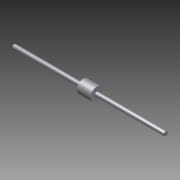
# Autodesk Inventor part: 042-DXDE0_rod
Saved by Autodesk Inventor 2012 (Build 160160000, 160)
## iProperties
Created: 2013-01-17
Part Number: 042-DXDE0_rod
Material: Default
Catalog Web Link: www.cadenas.de
Description: Standard Air Cylinder_rod-Original Line - Standard Air Cylinders
Vendor: BIMBA
Document SubType Name: Modeling
Designer: William
Manufacturer: BIMBA
Density: 1 g/cm^3
Category: PARTsolutions
Company: BIMBA
Title: 042-DXDE0_rod
Author: Cadenas PARTsolutions
Comments: Original Line - Standard Air Cylinders
PSOL_IDENT_0: {\\10.0.0.242\data_v9\23d-libs\bimba\bimba\bimba_imperial\bimba_full_line\original_line_cylinders\st
PSOL_IDENT_1: andard_air_cylinders\rod.prj},280 {VTYP=3D},{NB=042-DXDE0_rod},{LINA=042-DXDE0_rod},{NN=Standard Air
PSOL_IDENT_2: Cylinder_rod},{DATE=11.09.2012 07:37:40},{GEOMDATE=06.09.2012 09:06:00},{VERSION=},{LINEID=50},{LIN
PSOL_IDENT_3: ESUBID=-1},{WBVAR=STROKE,ACTING,MNT,DER,NR,BM,CO,M,EE,EEL,K,Q,Y,F,G,T,B,H,SER,SR,NT,W,E,HL,ST,STP,PR
PSOL_IDENT_4: C,PB,COLOR1}  {NB=042-DXDE0_rod},{LINA=042-DXDE0_rod},{KT=DUMMY},{PN=042-DXDE},{DASH=-},{BORE=0.7500
PSOL_IDENT_5: 0000},{BOREPN=04},{STROKE=2.000},{STROKEALG=[0.001:50/0.001]},{STROKE1=2.000},{ACTING=D},{ACTINGALG=
PSOL_IDENT_6: '' , 'Single Acting' , 'R' , 'Reverse Single Acting' , 'D' , 'Double Acting' },{ACTINGPN=D},{MNT=X}
PSOL_IDENT_7: ,{MNTALG= '' , 'Front Nose Mounting' , 'P' , 'Rear Pivot Mounting' , 'XP' , 'Double End or Pivot Mou
PSOL_IDENT_8: nting' , 'X' , 'Double End Mounting' , 'BF' , 'Front Block Mounting' , 'BR' , 'Rear Block Mounting f
PSOL_IDENT_9: or Vertical Positioning' , 'BFT' , 'Front Block Trunnion Mounting' , 'BRT' , 'Rear Block Trunnion Mo
PSOL_IDENT_10: unting' },{TYPE=},{MNTPN=X},{DER=DE},{DERALG= 'DE' , 'With Double End Rod' },{NR=},{NRALG= '' , 'N/A
PSOL_IDENT_11: ' },{NRPN=},{BM=},{BMALG= '' , 'N/A' },{BMPN=},{CO=},{COALG= '' , 'N/A' },{M=},{MALG= '', 'Without M
PSOL_IDENT_12: agnet', 'M', 'With Magnet' },{EE=},{EEL=0},{EEMAX=48},{EEALG= '', 'Without Extra Extension', 'EE', '
PSOL_IDENT_13: With Extra Extension' },{EELALG=0},{EEPN=},{EEPN1=0.000},{K=},{KALG= '', 'Standard' , 'K' , 'Ports R
PSOL_IDENT_14: otated 90deg' },{KPN=},{Q=},{QALG= '' , 'Without Side Ported Rear Head' , 'Q' , 'With Side Ported Re
PSOL_IDENT_15: ar Head' },{QPN=},{Y=},{YALG= '' , 'N/A' },{YPN=},{F=},{FALG= '', 'Standard', 'F', 'Molycoated Body'
PSOL_IDENT_16: },{FPN=},{G=},{GPN=},{T=},{TALG= '' , 'Standard' , 'N' , 'Low Temperature' , 'V' , 'High Temperatur
PSOL_IDENT_17: e' },{NPN=},{VPN=},{B=},{BALG= '', 'Without Bumper' , 'B' , 'With Bumper' },{BPN=},{H=},{HALG= '', '
PSOL_IDENT_18: N/A' },{HPN=},{SER=},{SERALG= '' , 'Without Spring Return' , 'JS' , 'With Spring Return' },{SR=},{SR
PSOL_IDENT_19: ALG= 'C' , 'Carbon Steel Rod' , 'SR' , '303 Stainless Steel Rod' , '' , '303 Stainless Steel Rod1' }
PSOL_IDENT_20: ,{SRPN=},{SRCON=0},{NT=},{NTPN=},{W=},{WALG= '' , 'Without Wiper' , 'W' , 'With Wiper' },{WPN=},{E=}
PSOL_IDENT_21: ,{EALG= '' , 'Without Special Lube and Seals' , 'E' , 'With Special Lube and Seals' },{EPN=},{HL=},{
PSOL_IDENT_22: HLALG= '' , 'Wihout Low Pressure Hydraulic' , 'HL' , 'With Low Pressure Hydraulic' },{ST=},{STALG= '
PSOL_IDENT_23: ' , 'Without Switch Track' , 'T' , 'With Switch Track' },{STP=},{STPALG= '' , 'N/A' },{STPN=},{PRC=}
PSOL_IDENT_24: ,{PRCALG= '' , 'Without Piston Rod Clevis' , 'D-166-1' , 'With Piston Rod Clevis' },{PRCPN=},{PB=},{
PSOL_IDENT_25: PBALG= '' , 'Without Pivot Bracket' , 'D-167' , 'With Pivot Bracket' },{PBPN=},{TLEN=3.2570},{TEXT=0
PSOL_IDENT_26: .233333},{SPACE=0.133333},{FRAC=9.0000},{RGCON=},{RGDACCON=R},{RHCON=DX},{RHCONON=0},{RHACCON=},{FNU
PSOL_IDENT_27: TCON=1},{RNUTCON=1},{FNUTPN=D-9},{RNUTPN=D-9},{FNUTTRANS=0.0000},{RNUTTRANS=0.0000},{VHOLECON=0},{A1
PSOL_IDENT_28: =1.5940},{A1N=0.8750},{A1P=1.5940},{A1B=1.5940},{A4=0.2525},{A4N=0.3130},{A4P=0.2525},{A5=0.0300},{A
PSOL_IDENT_29: 1H=1.594},{A1NH=0.5310},{A1PH=1.5940},{A1BH=1.0940},{A1SH=1.2190},{A2H=0.2190},{A2NH=0.2190},{LENGTH
PSOL_IDENT_30: =4.0000},{LENGTH1=4.0000},{LENGTH2=0.0000},{MUL=2.0000},{MUL11=2.0000},{MUL22=5.3800},{MUL33=5.3800}
PSOL_IDENT_31: ,{MUL2=2.0000},{MUL211=2.0000},{MUL222=2.6900},{MUL233=2.6900},{SSS=4.0000},{RGLEN=1.3715},{RHLEN=1.
PSOL_IDENT_32: 3715},{SSS1=3.0000},{A13=1.3120},{THDLEN1=0.5000},{THD1=0.2500},{TAB=UNF},{THDLEN=0.5000},{THD=0.250
PSOL_IDENT_33: 0},{OD=0.7615},{RODL=4.9060},{PL=0.8120},{RODDIA=0.2500},{HEX=0.2500},{RODTRANS=2.0000},{G1=0.1250},
PSOL_IDENT_34: {ON=0},{G5=0.6250},{DERLEN=4.0940},{THOLE=0.0000},{WF=0.2200},{BADD=0.0000},{MADD=0.0000},{NVADD=0.0
PSOL_IDENT_35: 00},{JRADD=0.00000},{COLOR=0.71,0.71,0.71,0.00},{GROOVE=1},{HOL=0},{D7=0.2520},{H1=1.1175},{D1=0.862
PSOL_IDENT_36: 5},{D1RH=0.8625},{D1P=0.8325},{D1B=0.8625},{D1N=0.8050},{D1NRH=0.8050},{D1BRH=0.8325},{D1PRH=0.8625}
PSOL_IDENT_37: ,{BOZO=0},{HADD=0.000},{COLOR1=0},{DEFL=0.0000},{HEXL=0.0000},{SSADD=0.0000},{WFL=0.0000},{MOVE=0.00
PSOL_IDENT_38: 00}
CNS_NT: Standard
CNS_NB: 042-DXDE0_rod
CNS_NBSYN: $PN.$COLOR1._rod
CNS_LINA: 042-DXDE0_rod
CNS_PN: 042-DXDE
CNS_DASH: -
CNS_BORE: 0.75000000
CNS_BOREPN: 04
CNS_STROKE: 2.000
CNS_STROKEALG: [0.001:50/0.001]
CNS_STROKE1: 2.000
CNS_ACTING: Double Acting
CNS_ACTINGALG: '' , 'Single Acting' , 'R' , 'Reverse Single Acting' , 'D' , 'Double Acting'
CNS_ACTINGPN: D
CNS_MNT: Double End Mounting
CNS_MNTALG: '' , 'Front Nose Mounting' , 'P' , 'Rear Pivot Mounting' , 'XP' , 'Double End or Pivot Mounting' , 'X' , 'Double End Mounting' , 'BF' , 'Front Block Mounting' , 'BR' , 'Rear Block Mounting for Vertical Positioning' , 'BFT' , 'Front Block Trunnion Mounting' , 'BRT' , 'Rear Block Trunnion Mounting'
CNS_MNTPN: X
CNS_DER: With Double End Rod
CNS_DERALG: 'DE' , 'With Double End Rod'
CNS_NR: N/A
CNS_NRALG: '' , 'N/A'
CNS_BM: N/A
CNS_BMALG: '' , 'N/A'
CNS_CO: N/A
CNS_COALG: '' , 'N/A'
CNS_M: Without Magnet
CNS_MALG: '', 'Without Magnet', 'M', 'With Magnet'
CNS_EE: Without Extra Extension
CNS_EEL: 0
CNS_EEMAX: 48
CNS_EEALG: '', 'Without Extra Extension', 'EE', 'With Extra Extension'
CNS_EELALG: 0
CNS_EEPN1: 0.000
CNS_K: Standard
CNS_KALG: '', 'Standard' , 'K' , 'Ports Rotated 90deg'
CNS_Q: Without Side Ported Rear Head
CNS_QALG: '' , 'Without Side Ported Rear Head' , 'Q' , 'With Side Ported Rear Head'
CNS_Y: N/A
CNS_YALG: '' , 'N/A'
CNS_F: Standard
CNS_FALG: '', 'Standard', 'F', 'Molycoated Body'
CNS_G: Without Magnalube Lubrication
CNS_T: Standard
CNS_TALG: '' , 'Standard' , 'N' , 'Low Temperature' , 'V' , 'High Temperature'
CNS_B: Without Bumper
CNS_BALG: '', 'Without Bumper' , 'B' , 'With Bumper'
CNS_H: N/A
CNS_HALG: '', 'N/A'
CNS_SER: Without Spring Return
CNS_SERALG: '' , 'Without Spring Return' , 'JS' , 'With Spring Return'
CNS_SR: 303 Stainless Steel Rod1
CNS_SRALG: 'C' , 'Carbon Steel Rod' , 'SR' , '303 Stainless Steel Rod' , '' , '303 Stainless Steel Rod1'
CNS_SRCON: 0
CNS_W: Without Wiper
CNS_WALG: '' , 'Without Wiper' , 'W' , 'With Wiper'
CNS_E: Without Special Lube and Seals
CNS_EALG: '' , 'Without Special Lube and Seals' , 'E' , 'With Special Lube and Seals'
CNS_HL: Wihout Low Pressure Hydraulic
CNS_HLALG: '' , 'Wihout Low Pressure Hydraulic' , 'HL' , 'With Low Pressure Hydraulic'
CNS_ST: Without Switch Track
CNS_STALG: '' , 'Without Switch Track' , 'T' , 'With Switch Track'
CNS_STP: N/A
CNS_STPALG: '' , 'N/A'
CNS_PRC: Without Piston Rod Clevis
CNS_PRCALG: '' , 'Without Piston Rod Clevis' , 'D-166-1' , 'With Piston Rod Clevis'
CNS_PB: Without Pivot Bracket
CNS_PBALG: '' , 'Without Pivot Bracket' , 'D-167' , 'With Pivot Bracket'
CNS_TLEN: 3.2570
CNS_TEXT: 0.233
CNS_SPACE: 0.133
CNS_FRAC: 9.0000
CNS_RGDACCON: R
CNS_RHCON: DX
CNS_RHCONON: 0
CNS_FNUTCON: 1
CNS_RNUTCON: 1
CNS_FNUTPN: D-9
CNS_RNUTPN: D-9
CNS_FNUTTRANS: 0.0000
CNS_RNUTTRANS: 0.0000
CNS_VHOLECON: 0
CNS_A1: 1.5940
CNS_A1N: 0.8750
CNS_A1P: 1.5940
CNS_A1B: 1.5940
CNS_A4: 0.2525
CNS_A4N: 0.3130
CNS_A4P: 0.2525
CNS_A5: 0.0300
CNS_A1H: 1.594
CNS_A1NH: 0.5310
CNS_A1PH: 1.5940
CNS_A1BH: 1.0940
CNS_A1SH: 1.2190
CNS_A2H: 0.2190
CNS_A2NH: 0.2190
CNS_LENGTH: 4.0000
CNS_LENGTH1: 4.0000
CNS_LENGTH2: 0.0000
CNS_MUL: 2.0000
CNS_MUL11: 2.0000
CNS_MUL22: 5.3800
CNS_MUL33: 5.3800
CNS_MUL2: 2.0000
CNS_MUL211: 2.0000
CNS_MUL222: 2.6900
CNS_MUL233: 2.6900
CNS_SSS: 4.0000
CNS_RGLEN: 1.3715
CNS_RHLEN: 1.3715
CNS_SSS1: 3.0000
CNS_A13: 1.3120
CNS_THDLEN1: 0.5000
CNS_THD1: 0.2500
CNS_TAB: UNF
CNS_THDLEN: 0.5000
CNS_THD: 0.2500
CNS_OD: 0.7615
CNS_RODL: 4.9060
CNS_PL: 0.8120
CNS_RODDIA: 0.2500
CNS_HEX: 0.2500
CNS_RODTRANS: 2.0000
CNS_G1: 0.1250
CNS_ON: 0
CNS_G5: 0.6250
CNS_DERLEN: 4.0940
CNS_THOLE: 0.0000
CNS_WF: 0.2200
CNS_BADD: 0.0000
CNS_MADD: 0.0000
CNS_NVADD: 0.000
CNS_JRADD: 0.00000
CNS_COLOR: 0.71,0.71,0.71,0.00
CNS_GROOVE: 1
CNS_HOL: 0
CNS_D7: 0.2520
CNS_H1: 1.1175
CNS_D1: 0.8625
CNS_D1RH: 0.8625
CNS_D1P: 0.8325
CNS_D1B: 0.8625
CNS_D1N: 0.8050
CNS_D1NRH: 0.8050
CNS_D1BRH: 0.8325
CNS_D1PRH: 0.8625
CNS_BOZO: 0
CNS_HADD: 0.000
CNS_COLOR1: 0
CNS_DEFL: 0.0000
CNS_HEXL: 0.0000
CNS_SSADD: 0.0000
CNS_WFL: 0.0000
CNS_MOVE: 0.0000
SUPPLIER: BIMBA
ARTICLENO: 042-DXDE0_rod
BOMINFO: 042-DXDE0_rod
CREATOR: CADENAS GmbH
Autodesk Inventor part; units mm, degrees
sketch "Sketch_1" plane through (0, 0, 0) normal (0, 0, 1) x (1, 0, 0)
  line L0 (111.9124, 0) -> (0, 0)
  line L1 (0, 0) -> (0, 3.175)
  line L2 (0, 3.175) -> (91.2876, 3.175)
  line L3 (91.2876, 3.175) -> (91.2876, 9.6203)
  line L4 (91.2876, 9.6203) -> (111.9124, 9.6203)
  line L5 (111.9124, 9.6203) -> (111.9124, 0)
  line L6 (111.9124, 0) -> (0, 0)
  constraints: 14 end point
revolve "Revolution1" add sketch "Sketch_1" angle 360 about axis through (111.9124, 0, 0) along (1, 0, 0)
sketch "Sketch_3" plane through (0, 0, 0) normal (0, 0, 1) x (1, 0, 0)
  line L0 (0, 0) -> (-12.7, 0)
  line L1 (-12.7, 0) -> (-12.7, 2.634)
  line L2 (-12.7, 2.634) -> (-12.159, 3.175)
  line L3 (-12.159, 3.175) -> (0, 3.175)
  line L4 (0, 3.175) -> (0, 0)
  line L5 (0, 0) -> (-12.7, 0)
  constraints: 12 end point
revolve "Revolution2" add sketch "Sketch_3" angle 360 about axis through (0, 0, 0) along (1, 0, 0)
sketch "Sketch_6" plane through (0, 0, 0) normal (0, 0, 1) x (1, 0, 0)
  line L0 (203.2, 0) -> (111.9124, 0)
  line L1 (111.9124, 0) -> (111.9124, 3.175)
  line L2 (111.9124, 3.175) -> (203.2, 3.175)
  line L3 (203.2, 3.175) -> (203.2, 0)
  line L4 (203.2, 0) -> (111.9124, 0)
  constraints: 10 end point
revolve "Revolution3" add sketch "Sketch_6" angle 360 about axis through (203.2, 0, 0) along (1, 0, 0)
sketch "Sketch_7" plane through (0, 0, 0) normal (0, 0, 1) x (1, 0, 0)
  line L0 (215.9, 0) -> (203.2, 0)
  line L1 (203.2, 0) -> (203.2, 3.175)
  line L2 (203.2, 3.175) -> (215.359, 3.175)
  line L3 (215.359, 3.175) -> (215.9, 2.634)
  line L4 (215.9, 2.634) -> (215.9, 0)
  line L5 (215.9, 0) -> (203.2, 0)
  constraints: 12 end point
revolve "Revolution4" add sketch "Sketch_7" angle 360 about axis through (215.9, 0, 0) along (1, 0, 0)
sketch "Sketch_30" plane through (0, 0, 0) normal (0, 0, 1) x (1, 0, 0)
  line L0 (0, 0) -> (-0.254, 0)
  line L1 (-0.254, 3.429) -> (-0.254, 2.921)
  line L2 (-0.254, 2.921) -> (0, 2.921)
  line L3 (0, 2.921) -> (0, 3.429)
  line L4 (0, 3.429) -> (-0.254, 3.429)
  constraints: 10 end point
revolve "Revolution5" cut sketch "Sketch_30" angle 360 about axis through (0, 0, 0) along (1, 0, 0)
sketch "Sketch_40" plane through (0, 0, 0) normal (0, 0, 1) x (1, 0, 0)
  line L0 (203.454, 0) -> (203.2, 0)
  line L1 (203.2, 3.429) -> (203.2, 2.921)
  line L2 (203.2, 2.921) -> (203.454, 2.921)
  line L3 (203.454, 2.921) -> (203.454, 3.429)
  line L4 (203.454, 3.429) -> (203.2, 3.429)
  constraints: 10 end point
revolve "Revolution6" cut sketch "Sketch_40" angle 360 about axis through (203.454, 0, 0) along (1, 0, 0)
ref_plane "rod_cp_XY" through (0, 0, 0) normal (1, 0, 0) x (0, 0, -1)
ref_plane "rod_cp_YZ" through (0, 0, 0) normal (0, 0, -1) x (0, 1, 0)
ref_plane "rod_cp_ZX" through (0, 0, 0) normal (0, 1, 0) x (1, 0, 0)
ref_plane "to_rod_clevis_XY" through (-12.7, 0, 0) normal (1, 0, 0) x (0, 0, -1)
ref_plane "to_rod_clevis_YZ" through (-12.7, 0, 0) normal (0, 0, -1) x (0, 1, 0)
ref_plane "to_rod_clevis_ZX" through (-12.7, 0, 0) normal (0, 1, 0) x (1, 0, 0)
ref_plane "rl2_XY" through (0, 0, 0) normal (1, 0, 0) x (0, 0, -1)
ref_plane "rl2_YZ" through (0, 0, 0) normal (0, 0, -1) x (0, 1, 0)
ref_plane "rl2_ZX" through (0, 0, 0) normal (0, 1, 0) x (1, 0, 0)
ref_plane "rl1_XY" through (-12.7, 0, 0) normal (1, 0, 0) x (0, 0, -1)
ref_plane "rl1_YZ" through (-12.7, 0, 0) normal (0, 0, -1) x (0, 1, 0)
ref_plane "rl1_ZX" through (-12.7, 0, 0) normal (0, 1, 0) x (1, 0, 0)
ref_plane "rl1_der_XY" through (215.9, 0, 0) normal (1, 0, 0) x (0, 0, -1)
ref_plane "rl1_der_YZ" through (215.9, 0, 0) normal (0, 0, -1) x (0, 1, 0)
ref_plane "rl1_der_ZX" through (215.9, 0, 0) normal (0, 1, 0) x (1, 0, 0)
ref_plane "rl2_der_XY" through (203.2, 0, 0) normal (1, 0, 0) x (0, 0, -1)
ref_plane "rl2_der_YZ" through (203.2, 0, 0) normal (0, 0, -1) x (0, 1, 0)
ref_plane "rl2_der_ZX" through (203.2, 0, 0) normal (0, 1, 0) x (1, 0, 0)
ref_plane "thd1_XY" through (-12.7, 3.175, 0) normal (1, 0, 0) x (0, 0, -1)
ref_plane "thd1_YZ" through (-12.7, 3.175, 0) normal (0, 0, -1) x (0, 1, 0)
ref_plane "thd1_ZX" through (-12.7, 3.175, 0) normal (0, 1, 0) x (1, 0, 0)
ref_plane "thd2_XY" through (-12.7, -3.175, 0) normal (1, 0, 0) x (0, 0, -1)
ref_plane "thd2_YZ" through (-12.7, -3.175, 0) normal (0, 0, -1) x (0, 1, 0)
ref_plane "thd2_ZX" through (-12.7, -3.175, 0) normal (0, 1, 0) x (1, 0, 0)
ref_plane "dia1_XY" through (0, 3.175, 0) normal (1, 0, 0) x (0, 0, -1)
ref_plane "dia1_YZ" through (0, 3.175, 0) normal (0, 0, -1) x (0, 1, 0)
ref_plane "dia1_ZX" through (0, 3.175, 0) normal (0, 1, 0) x (1, 0, 0)
ref_plane "dia2_XY" through (0, -3.175, 0) normal (1, 0, 0) x (0, 0, -1)
ref_plane "dia2_YZ" through (0, -3.175, 0) normal (0, 0, -1) x (0, 1, 0)
ref_plane "dia2_ZX" through (0, -3.175, 0) normal (0, 1, 0) x (1, 0, 0)
ref_plane "stroke1_XY" through (0, 0, 0) normal (1, 0, 0) x (0, 0, -1)
ref_plane "stroke1_YZ" through (0, 0, 0) normal (0, 0, -1) x (0, 1, 0)
ref_plane "stroke1_ZX" through (0, 0, 0) normal (0, 1, 0) x (1, 0, 0)
ref_plane "dia12_XY" through (0, 0, 10.9537) normal (1, 0, 0) x (0, 0, -1)
ref_plane "dia12_YZ" through (0, 0, 10.9537) normal (0, 0, -1) x (0, 1, 0)
ref_plane "dia12_ZX" through (0, 0, 10.9537) normal (0, 1, 0) x (1, 0, 0)
ref_plane "dia22_XY" through (0, 0, -10.9537) normal (1, 0, 0) x (0, 0, -1)
ref_plane "dia22_YZ" through (0, 0, -10.9537) normal (0, 0, -1) x (0, 1, 0)
ref_plane "dia22_ZX" through (0, 0, -10.9537) normal (0, 1, 0) x (1, 0, 0)
body "Solid1"
